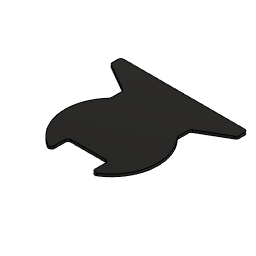
キッカー基板 (Autodesk Fusion 360 design; units mm, degrees)
Autodesk Fusion 360 part; units mm, degrees
note: some values were not read from the file. Set by a fixed rule: which sketch regions a step uses.
(part 1 of 4)
sketch "スケッチ1" plane through (0, 0, 0) normal (0, 0, 1) x (1, 0, 0)
  circle A0 centre (0, 0) radius 104
  line L0 (0, 0) -> (90.0666, 52)
  line L1 (0, 0) -> (104, 0) construction
  dimension "d1" = 208
  dimension "d2" = 30
  constraint coincident A0.centre L0.start
  constraint horizontal L1
  constraint coincident A0 L0.end
  measures "d1" diameter of A0
  measures "d2" angle of L0 L1
extrude "押し出し1" add sketch "スケッチ1" along normal blind 1.5 makes body 1
sketch "スケッチ2" plane through (0, 0, 1.5) normal (0, 0, 1) x (-1, 0, 0)
sketch "スケッチ3" plane through (0, 0, 3) normal (0, 0, 1) x (1, 0, 0)
  circle A0 centre (-65.4951, 21.3591) radius 1.5
  line L0 (-68.4502, 26.2407) -> (-71.2002, 21.4776)
  line L1 (-71.2002, 21.4776) -> (-64.272, 17.4776)
  line L2 (-64.272, 17.4776) -> (-61.522, 22.2407)
  line L3 (-61.522, 22.2407) -> (-68.4502, 26.2407)
sketch "スケッチ4" plane through (0, 0, 3) normal (0, 0, 1) x (1, 0, 0)
  circle A0 centre (65.4951, 21.3591) radius 1.5
  line L0 (71.2002, 21.4776) -> (68.4502, 26.2407)
  line L1 (68.4502, 26.2407) -> (61.522, 22.2407)
  line L2 (61.522, 22.2407) -> (64.272, 17.4776)
  line L3 (64.272, 17.4776) -> (71.2002, 21.4776)
sketch "スケッチ5" plane through (0, 0, 3) normal (0, 0, 1) x (1, 0, 0)
  circle A0 centre (-37.5827, -57.7353) radius 1.5
  line L0 (-43.0628, -59.3263) -> (-39.1737, -63.2153)
  line L1 (-39.1737, -63.2153) -> (-33.5169, -57.5585)
  line L2 (-33.5169, -57.5585) -> (-37.4059, -53.6694)
  line L3 (-37.4059, -53.6694) -> (-43.0628, -59.3263)
sketch "スケッチ6" plane through (0, 0, 3) normal (0, 0, 1) x (1, 0, 0)
  circle A0 centre (51.2451, 46.0409) radius 1.5
  line L0 (56.9502, 46.1593) -> (54.2002, 50.9224)
  line L1 (54.2002, 50.9224) -> (47.272, 46.9224)
  line L2 (47.272, 46.9224) -> (50.022, 42.1593)
  line L3 (50.022, 42.1593) -> (56.9502, 46.1593)
sketch "スケッチ7" plane through (0, 0, 3) normal (0, 0, 1) x (1, 0, 0)
  circle A0 centre (-51.2451, 46.0409) radius 1.5
  line L0 (-54.2002, 50.9224) -> (-56.9502, 46.1593)
  line L1 (-56.9502, 46.1593) -> (-50.022, 42.1593)
  line L2 (-50.022, 42.1593) -> (-47.272, 46.9224)
  line L3 (-47.272, 46.9224) -> (-54.2002, 50.9224)
sketch "スケッチ8" plane through (0, 0, 3) normal (0, 0, 1) x (1, 0, 0)
  circle A0 centre (-57.7353, -37.5827) radius 1.5
  line L0 (-63.2153, -39.1737) -> (-59.3263, -43.0628)
  line L1 (-59.3263, -43.0628) -> (-53.6694, -37.4059)
  line L2 (-53.6694, -37.4059) -> (-57.5585, -33.5169)
  line L3 (-57.5585, -33.5169) -> (-63.2153, -39.1737)
sketch "スケッチ9" plane through (0, 0, 3) normal (0, 0, 1) x (1, 0, 0)
  circle A0 centre (37.5827, -57.7353) radius 1.5
  line L0 (39.1737, -63.2153) -> (43.0628, -59.3263)
  line L1 (43.0628, -59.3263) -> (37.4059, -53.6694)
  line L2 (37.4059, -53.6694) -> (33.5169, -57.5585)
  line L3 (33.5169, -57.5585) -> (39.1737, -63.2153)
sketch "スケッチ10" plane through (0, 0, 3) normal (0, 0, 1) x (1, 0, 0)
  circle A0 centre (57.7353, -37.5827) radius 1.5
  line L0 (59.3263, -43.0628) -> (63.2153, -39.1737)
  line L1 (63.2153, -39.1737) -> (57.5585, -33.5169)
  line L2 (57.5585, -33.5169) -> (53.6694, -37.4059)
  line L3 (53.6694, -37.4059) -> (59.3263, -43.0628)
extrude "押し出し2" cut sketch "スケッチ7" against normal blind 10 contours A0 bodies 1
extrude "押し出し3" cut sketch "スケッチ6" against normal blind 4 contours A0 bodies 1
extrude "押し出し4" cut sketch "スケッチ3" against normal blind 6 contours A0 bodies 1
extrude "押し出し5" cut sketch "スケッチ8" against normal blind 13 contours A0 bodies 1
extrude "押し出し6" cut sketch "スケッチ5" against normal blind 16 contours A0 bodies 1
extrude "押し出し7" cut sketch "スケッチ9" against normal blind 5 contours A0 bodies 1
extrude "押し出し8" cut sketch "スケッチ10" against normal blind 12 contours A0 bodies 1
extrude "押し出し9" cut sketch "スケッチ4" against normal blind 13 contours A0 bodies 1
sketch "スケッチ11" plane through (0, 0, 0) normal (0, 0, -1) x (1, 0, 0)
  circle A0 centre (65.4951, -21.3591) radius 1.5
  circle A1 centre (57.7353, 37.5827) radius 1.5
  circle A2 centre (37.5827, 57.7353) radius 1.5
  circle A3 centre (-37.5827, 57.7353) radius 1.5
  circle A4 centre (-57.7353, 37.5827) radius 1.5
  circle A5 centre (-65.4951, -21.3591) radius 1.5
  circle A6 centre (51.2451, -46.0409) radius 1.5
  circle A7 centre (-51.2451, -46.0409) radius 1.5
  circle A8 centre (0, 0) radius 104
  line L0 (51.2451, -46.0409) -> (65.4951, -21.3591)
  line L1 (-65.4951, -21.3591) -> (-51.2451, -46.0409)
  line L2 (37.5827, 57.7353) -> (57.7353, 37.5827)
  line L3 (-57.7353, 37.5827) -> (-37.5827, 57.7353)
  line L4 (58.3701, -33.7) -> (69.6284, -40.2)
  line L5 (-58.3701, -33.7) -> (-69.6284, -40.2)
  line L6 (47.659, 47.659) -> (56.8514, 56.8514)
  line L7 (-47.659, 47.659) -> (-56.8514, 56.8514)
  line L8 (-56.8514, 56.8514) -> (-35.6382, 78.0646)
  line L9 (-56.8514, 56.8514) -> (-78.0646, 35.6382)
  line L10 (-78.0646, 35.6382) -> (-91.6263, 49.1999)
  line L11 (-35.6382, 78.0646) -> (-49.1999, 91.6263)
  line L12 (56.8514, 56.8514) -> (35.6382, 78.0646)
  line L13 (56.8514, 56.8514) -> (78.0646, 35.6382)
  line L14 (78.0646, 35.6382) -> (91.6263, 49.1999)
  line L15 (35.6382, 78.0646) -> (49.1999, 91.6263)
  line L16 (69.6284, -40.2) -> (84.6284, -14.2192)
  line L17 (84.6284, -14.2192) -> (101.238, -23.8088)
  line L18 (69.6284, -40.2) -> (54.6284, -66.1808)
  line L19 (54.6284, -66.1808) -> (71.238, -75.7703)
  line L20 (-69.6284, -40.2) -> (-54.6284, -66.1808)
  line L21 (-69.6284, -40.2) -> (-84.6284, -14.2192)
  line L22 (-84.6284, -14.2192) -> (-101.238, -23.8088)
  line L23 (-54.6284, -66.1808) -> (-71.238, -75.7703)
  dimension "d26" = 13
  dimension "d27" = 13
  dimension "d28" = 13
  dimension "d29" = 13
  dimension "d30" = 30
  dimension "d31" = 30
  dimension "d32" = 30
  dimension "d33" = 30
  dimension "d34" = 30
  dimension "d35" = 30
  dimension "d36" = 30
  dimension "d37" = 30
  constraint coincident A6.centre L0.start
  constraint coincident A0.centre L0.end
  constraint coincident A5.centre L1.start
  constraint coincident A7.centre L1.end
  constraint coincident A2.centre L2.start
  constraint coincident A1.centre L2.end
  constraint coincident A4.centre L3.start
  constraint coincident A3.centre L3.end
  constraint midpoint L0 L4.start
  constraint perpendicular L0 L4
  constraint midpoint L1 L5.start
  constraint perpendicular L1 L5
  constraint midpoint L2 L6.start
  constraint perpendicular L2 L6
  constraint midpoint L3 L7.start
  constraint perpendicular L3 L7
  constraint perpendicular L7 L8
  constraint perpendicular L7 L9
  constraint coincident A8 L10.end
  constraint perpendicular L9 L10
  constraint coincident A8 L11.end
  constraint perpendicular L8 L11
  constraint perpendicular L6 L12
  constraint perpendicular L6 L13
  constraint coincident A8 L14.end
  constraint perpendicular L13 L14
  constraint coincident A8 L15.end
  constraint perpendicular L12 L15
  constraint perpendicular L4 L16
  constraint coincident A8 L17.end
  constraint perpendicular L16 L17
  constraint perpendicular L4 L18
  constraint coincident A8 L19.end
  constraint perpendicular L18 L19
  constraint perpendicular L5 L20
  constraint perpendicular L5 L21
  constraint coincident A8 L22.end
  constraint perpendicular L21 L22
  constraint coincident A8 L23.end
  constraint perpendicular L20 L23
  measures "d26" distance of L4.start L4.end
  measures "d27" distance of L5.start L5.end
  measures "d28" distance of L6.start L6.end
  measures "d29" distance of L7.start L7.end
  measures "d30" distance of L7.end L8.end
  measures "d31" distance of L7.end L9.end
  measures "d32" distance of L6.end L12.end
  measures "d33" distance of L6.end L13.end
  measures "d34" distance of L4.end L16.end
  measures "d35" distance of L4.end L18.end
  measures "d36" distance of L5.end L20.end
  measures "d37" distance of L5.end L21.end
extrude "押し出し10" cut sketch "スケッチ11" against normal blind 40 contours A8 L12 L13 L14 L15 | A8 L16 L17 L18 L19 | A8 L8 L9 L10 L11 | A8 L20 L21 L22 L23 bodies 1
move_body "移動1" bodies 1 to x (-1, 0, 0) y (0, 1, 0) z (0, 0, -1) at (0, 0, 3)
sketch "スケッチ12" plane through (0, 0, 3) normal (0, 0, 1) x (-1, 0, 0)
  line L0 (35.6382, 78.0646) -> (49.1999, 91.6263)
  arc A0 (49.1999, 91.6263) -> (-49.1999, 91.6263) centre (0, 0) ccw
  line L1 (-49.1999, 91.6263) -> (-35.6382, 78.0646)
  line L2 (-35.6382, 78.0646) -> (-78.0646, 35.6382)
  line L3 (-78.0646, 35.6382) -> (-91.6263, 49.1999)
  arc A1 (-91.6263, 49.1999) -> (-101.238, -23.8088) centre (0, 0) ccw
  line L4 (-101.238, -23.8088) -> (-84.6284, -14.2192)
  line L5 (-84.6284, -14.2192) -> (-54.6284, -66.1808)
  line L6 (-54.6284, -66.1808) -> (-71.238, -75.7703)
  arc A2 (-71.238, -75.7703) -> (71.238, -75.7703) centre (0, 0) ccw
  line L7 (71.238, -75.7703) -> (54.6284, -66.1808)
  line L8 (54.6284, -66.1808) -> (84.6284, -14.2192)
  line L9 (84.6284, -14.2192) -> (101.238, -23.8088)
  arc A3 (101.238, -23.8088) -> (91.6263, 49.1999) centre (0, 0) ccw
  line L10 (91.6263, 49.1999) -> (78.0646, 35.6382)
  line L11 (78.0646, 35.6382) -> (35.6382, 78.0646)
  circle A4 centre (65.4951, -21.3591) radius 1.5
  circle A5 centre (57.7353, 37.5827) radius 1.5
  circle A6 centre (37.5827, 57.7353) radius 1.5
  circle A7 centre (-37.5827, 57.7353) radius 1.5
  circle A8 centre (-57.7353, 37.5827) radius 1.5
  circle A9 centre (-65.4951, -21.3591) radius 1.5
  circle A10 centre (51.2451, -46.0409) radius 1.5
  circle A11 centre (-51.2451, -46.0409) radius 1.5
  line L12 (0, -104) -> (0, -64)
  line L13 (0, -64) -> (-40, -64)
  line L14 (-40, -64) -> (-40, -96)
  line L15 (0, -64) -> (40, -64)
  line L16 (40, -64) -> (40, -96)
  dimension "d40" = 40
  constraint midpoint A2 L12.start
  constraint vertical L12
  constraint perpendicular L12 L13
  constraint coincident A2 L14.end
  constraint perpendicular L13 L14
  constraint perpendicular L14 L15
  constraint coincident A2 L16.end
  constraint perpendicular L15 L16
  measures "d40" distance of L12.start L12.end
extrude "押し出し11" cut sketch "スケッチ12" against normal blind 35 contours A2 L12 L15 L16 | A2 L12 L13 L14 bodies 1
sketch "スケッチ13" plane through (0, 0, 3) normal (0, 0, 1) x (-1, 0, 0)
  line L0 (40, -64) -> (40, -96)
  arc A0 (40, -96) -> (71.238, -75.7703) centre (0, 0) ccw
  line L1 (71.238, -75.7703) -> (54.6284, -66.1808)
  line L2 (54.6284, -66.1808) -> (84.6284, -14.2192)
  line L3 (84.6284, -14.2192) -> (101.238, -23.8088)
  arc A1 (101.238, -23.8088) -> (91.6263, 49.1999) centre (0, 0) ccw
  line L4 (91.6263, 49.1999) -> (78.0646, 35.6382)
  line L5 (78.0646, 35.6382) -> (35.6382, 78.0646)
  line L6 (35.6382, 78.0646) -> (49.1999, 91.6263)
  arc A2 (49.1999, 91.6263) -> (-49.1999, 91.6263) centre (0, 0) ccw
  line L7 (-49.1999, 91.6263) -> (-35.6382, 78.0646)
  line L8 (-35.6382, 78.0646) -> (-78.0646, 35.6382)
  line L9 (-78.0646, 35.6382) -> (-91.6263, 49.1999)
  arc A3 (-91.6263, 49.1999) -> (-101.238, -23.8088) centre (0, 0) ccw
  line L10 (-101.238, -23.8088) -> (-84.6284, -14.2192)
  line L11 (-84.6284, -14.2192) -> (-54.6284, -66.1808)
  line L12 (-54.6284, -66.1808) -> (-71.238, -75.7703)
  arc A4 (-71.238, -75.7703) -> (-40, -96) centre (0, 0) ccw
  line L13 (-40, -96) -> (-40, -64)
  line L14 (-40, -64) -> (40, -64)
  circle A5 centre (65.4951, -21.3591) radius 1.5
  circle A6 centre (57.7353, 37.5827) radius 1.5
  circle A7 centre (37.5827, 57.7353) radius 1.5
  circle A8 centre (-37.5827, 57.7353) radius 1.5
  circle A9 centre (-57.7353, 37.5827) radius 1.5
  circle A10 centre (-65.4951, -21.3591) radius 1.5
  circle A11 centre (51.2451, -46.0409) radius 1.5
  circle A12 centre (-51.2451, -46.0409) radius 1.5
  line L15 (-40, -64) -> (-40, -84)
  line L16 (-40, -84) -> (-61.3188, -84)
  line L17 (40, -84.2208) -> (61.0153, -84.2208)
  dimension "d43" = 20
  constraint coincident L13.end L14.start
  constraint perpendicular L14 L15
  constraint coincident A4 L16.end
  constraint perpendicular L13 L16
  constraint coincident L0 L17.start
  constraint coincident A0 L17.end
  constraint perpendicular L0 L17
  measures "d43" distance of L13.end L15.end
extrude "押し出し12" cut sketch "スケッチ13" against normal blind 18 contours L0 A0 L17 | A4 L13 L16 bodies 1
sketch "スケッチ14" plane through (0, 0, 3) normal (0, 0, 1) x (-1, 0, 0)
  line L0 (40, -84.2208) -> (61.0153, -84.2208)
  arc A0 (61.0153, -84.2208) -> (71.238, -75.7703) centre (0, 0) ccw
  line L1 (71.238, -75.7703) -> (54.6284, -66.1808)
  line L2 (54.6284, -66.1808) -> (84.6284, -14.2192)
  line L3 (84.6284, -14.2192) -> (101.238, -23.8088)
  arc A1 (101.238, -23.8088) -> (91.6263, 49.1999) centre (0, 0) ccw
  line L4 (91.6263, 49.1999) -> (78.0646, 35.6382)
  line L5 (78.0646, 35.6382) -> (35.6382, 78.0646)
  line L6 (35.6382, 78.0646) -> (49.1999, 91.6263)
  arc A2 (49.1999, 91.6263) -> (-49.1999, 91.6263) centre (0, 0) ccw
  line L7 (-49.1999, 91.6263) -> (-35.6382, 78.0646)
  line L8 (-35.6382, 78.0646) -> (-78.0646, 35.6382)
  line L9 (-78.0646, 35.6382) -> (-91.6263, 49.1999)
  arc A3 (-91.6263, 49.1999) -> (-101.238, -23.8088) centre (0, 0) ccw
  line L10 (-101.238, -23.8088) -> (-84.6284, -14.2192)
  line L11 (-84.6284, -14.2192) -> (-54.6284, -66.1808)
  line L12 (-54.6284, -66.1808) -> (-71.238, -75.7703)
  arc A4 (-71.238, -75.7703) -> (-61.3188, -84) centre (0, 0) ccw
  line L13 (-61.3188, -84) -> (-40, -84)
  line L14 (-40, -84) -> (-40, -64)
  line L15 (-40, -64) -> (40, -64)
  line L16 (40, -64) -> (40, -84.2208)
  circle A5 centre (65.4951, -21.3591) radius 1.5
  circle A6 centre (57.7353, 37.5827) radius 1.5
  circle A7 centre (37.5827, 57.7353) radius 1.5
  circle A8 centre (-37.5827, 57.7353) radius 1.5
  circle A9 centre (-57.7353, 37.5827) radius 1.5
  circle A10 centre (-65.4951, -21.3591) radius 1.5
  circle A11 centre (51.2451, -46.0409) radius 1.5
  circle A12 centre (-51.2451, -46.0409) radius 1.5
  circle A13 centre (0, 0) radius 50
  constraint coincident A0.centre A1.centre
extrude "押し出し13" cut sketch "スケッチ14" against normal blind 30 contours A13 bodies 1
sketch "スケッチ15" plane through (0, 0, 3) normal (0, 0, 1) x (-1, 0, 0)
  circle A0 centre (0, 0) radius 50
  line L0 (40, -84.2208) -> (61.0153, -84.2208)
  arc A1 (61.0153, -84.2208) -> (71.238, -75.7703) centre (0, 0) ccw
  line L1 (71.238, -75.7703) -> (54.6284, -66.1808)
  line L2 (54.6284, -66.1808) -> (84.6284, -14.2192)
  line L3 (84.6284, -14.2192) -> (101.238, -23.8088)
  arc A2 (101.238, -23.8088) -> (91.6263, 49.1999) centre (0, 0) ccw
  line L4 (91.6263, 49.1999) -> (78.0646, 35.6382)
  line L5 (78.0646, 35.6382) -> (35.6382, 78.0646)
  line L6 (35.6382, 78.0646) -> (49.1999, 91.6263)
  arc A3 (49.1999, 91.6263) -> (-49.1999, 91.6263) centre (0, 0) ccw
  line L7 (-49.1999, 91.6263) -> (-35.6382, 78.0646)
  line L8 (-35.6382, 78.0646) -> (-78.0646, 35.6382)
  line L9 (-78.0646, 35.6382) -> (-91.6263, 49.1999)
  arc A4 (-91.6263, 49.1999) -> (-101.238, -23.8088) centre (0, 0) ccw
  line L10 (-101.238, -23.8088) -> (-84.6284, -14.2192)
  line L11 (-84.6284, -14.2192) -> (-54.6284, -66.1808)
  line L12 (-54.6284, -66.1808) -> (-71.238, -75.7703)
  arc A5 (-71.238, -75.7703) -> (-61.3188, -84) centre (0, 0) ccw
  line L13 (-61.3188, -84) -> (-40, -84)
  line L14 (-40, -84) -> (-40, -64)
  line L15 (-40, -64) -> (40, -64)
  line L16 (40, -64) -> (40, -84.2208)
  circle A6 centre (65.4951, -21.3591) radius 1.5
  circle A7 centre (57.7353, 37.5827) radius 1.5
  circle A8 centre (37.5827, 57.7353) radius 1.5
  circle A9 centre (-37.5827, 57.7353) radius 1.5
  circle A10 centre (-57.7353, 37.5827) radius 1.5
  circle A11 centre (-65.4951, -21.3591) radius 1.5
  circle A12 centre (51.2451, -46.0409) radius 1.5
  circle A13 centre (-51.2451, -46.0409) radius 1.5
  circle A14 centre (0, 0) radius 42
  dimension "d48" = 84
  constraint coincident A0.centre A1.centre
  measures "d48" diameter of A14
extrude "押し出し14" add sketch "スケッチ15" against normal blind 1.5 separate body contours A14 makes body 2
sketch "スケッチ16" plane through (0, 0, 3) normal (0, 0, 1) x (-1, 0, 0)
  circle A0 centre (0, 0) radius 42
  circle A1 centre (0, 0) radius 37
  dimension "d51" = 74
  constraint concentric A0 A1
  measures "d51" diameter of A1
extrude "押し出し15" cut sketch "スケッチ16" against normal blind 25 contours A1 bodies 2
sketch "スケッチ17" plane through (0, 0, 3) normal (0, 0, 1) x (-1, 0, 0)
  circle A0 centre (0, 0) radius 50
  line L0 (40, -84.2208) -> (61.0153, -84.2208)
  arc A1 (61.0153, -84.2208) -> (71.238, -75.7703) centre (0, 0) ccw
  line L1 (71.238, -75.7703) -> (54.6284, -66.1808)
  line L2 (54.6284, -66.1808) -> (84.6284, -14.2192)
  line L3 (84.6284, -14.2192) -> (101.238, -23.8088)
  arc A2 (101.238, -23.8088) -> (91.6263, 49.1999) centre (0, 0) ccw
  line L4 (91.6263, 49.1999) -> (78.0646, 35.6382)
  line L5 (78.0646, 35.6382) -> (35.6382, 78.0646)
  line L6 (35.6382, 78.0646) -> (49.1999, 91.6263)
  arc A3 (49.1999, 91.6263) -> (-49.1999, 91.6263) centre (0, 0) ccw
  line L7 (-49.1999, 91.6263) -> (-35.6382, 78.0646)
  line L8 (-35.6382, 78.0646) -> (-78.0646, 35.6382)
  line L9 (-78.0646, 35.6382) -> (-91.6263, 49.1999)
  arc A4 (-91.6263, 49.1999) -> (-101.238, -23.8088) centre (0, 0) ccw
  line L10 (-101.238, -23.8088) -> (-84.6284, -14.2192)
  line L11 (-84.6284, -14.2192) -> (-54.6284, -66.1808)
  line L12 (-54.6284, -66.1808) -> (-71.238, -75.7703)
  arc A5 (-71.238, -75.7703) -> (-61.3188, -84) centre (0, 0) ccw
  line L13 (-61.3188, -84) -> (-40, -84)
  line L14 (-40, -84) -> (-40, -64)
  line L15 (-40, -64) -> (40, -64)
  line L16 (40, -64) -> (40, -84.2208)
  circle A6 centre (65.4951, -21.3591) radius 1.5
  circle A7 centre (57.7353, 37.5827) radius 1.5
  circle A8 centre (37.5827, 57.7353) radius 1.5
  circle A9 centre (-37.5827, 57.7353) radius 1.5
  circle A10 centre (-57.7353, 37.5827) radius 1.5
  circle A11 centre (-65.4951, -21.3591) radius 1.5
  circle A12 centre (51.2451, -46.0409) radius 1.5
  circle A13 centre (-51.2451, -46.0409) radius 1.5
  line L17 (0, -64) -> (0, -58)
  line L18 (0, -58) -> (-40, -58)
  line L19 (-40, -58) -> (-40, -50)
  line L20 (-40, -50) -> (0, -50)
  line L21 (0, -58) -> (40, -58)
  line L22 (40, -58) -> (40, -50)
  line L23 (40, -50) -> (0, -50)
  line L24 (-4, -50.1) -> (-4, -50)
  constraint midpoint L15 L17.start
  constraint perpendicular L15 L17
  constraint perpendicular L17 L18
  constraint perpendicular L18 L19
  constraint coincident A0 L20.end
  constraint tangent A0 L20
  constraint perpendicular L17 L21
  constraint perpendicular L21 L22
  constraint tangent A0 L23
  constraint coincident L20 L24.end
  constraint perpendicular L20 L24
extrude "押し出し16" cut sketch "スケッチ17" against normal blind 13 contours L18 L19 L20 L21 L22 L23 bodies 1
sketch "スケッチ18" plane through (0, 0, 3) normal (0, 0, 1) x (-1, 0, 0)
  circle A0 centre (-51.2451, -46.0409) radius 1.5
  circle A1 centre (51.2451, -46.0409) radius 1.5
  circle A2 centre (-65.4951, -21.3591) radius 1.5
  circle A3 centre (-57.7353, 37.5827) radius 1.5
  circle A4 centre (-37.5827, 57.7353) radius 1.5
  circle A5 centre (37.5827, 57.7353) radius 1.5
  circle A6 centre (57.7353, 37.5827) radius 1.5
  circle A7 centre (65.4951, -21.3591) radius 1.5
  line L0 (40, -84.2208) -> (61.0153, -84.2208)
  arc A8 (61.0153, -84.2208) -> (71.238, -75.7703) centre (0, 0) ccw
  line L1 (71.238, -75.7703) -> (54.6284, -66.1808)
  line L2 (54.6284, -66.1808) -> (84.6284, -14.2192)
  line L3 (84.6284, -14.2192) -> (101.238, -23.8088)
  arc A9 (101.238, -23.8088) -> (91.6263, 49.1999) centre (0, 0) ccw
  line L4 (91.6263, 49.1999) -> (78.0646, 35.6382)
  line L5 (78.0646, 35.6382) -> (35.6382, 78.0646)
  line L6 (35.6382, 78.0646) -> (49.1999, 91.6263)
  arc A10 (49.1999, 91.6263) -> (-49.1999, 91.6263) centre (0, 0) ccw
  line L7 (-49.1999, 91.6263) -> (-35.6382, 78.0646)
  line L8 (-35.6382, 78.0646) -> (-78.0646, 35.6382)
  line L9 (-78.0646, 35.6382) -> (-91.6263, 49.1999)
  arc A11 (-91.6263, 49.1999) -> (-101.238, -23.8088) centre (0, 0) ccw
  line L10 (-101.238, -23.8088) -> (-84.6284, -14.2192)
  line L11 (-84.6284, -14.2192) -> (-54.6284, -66.1808)
  line L12 (-54.6284, -66.1808) -> (-71.238, -75.7703)
  arc A12 (-71.238, -75.7703) -> (-61.3188, -84) centre (0, 0) ccw
  line L13 (-61.3188, -84) -> (-40, -84)
  line L14 (-40, -84) -> (-40, -64)
  line L15 (-40, -64) -> (40, -64)
  line L16 (40, -64) -> (40, -84.2208)
  circle A13 centre (0, 0) radius 50
  line L17 (0, -50) -> (40, -50)
  line L18 (40, -50) -> (40, -58)
  line L19 (40, -58) -> (-40, -58)
  line L20 (-40, -58) -> (-40, -50)
  line L21 (-40, -50) -> (0, -50)
  circle A14 centre (0, 0) radius 45
  circle A15 centre (0, 0) radius 371.5
  dimension "d56" = 743
  constraint coincident A8.centre A9.centre
  constraint concentric A8 A15
  measures "d56" diameter of A15
extrude "押し出し17" add sketch "スケッチ18" against normal blind 1.5 contours A13 bodies 1
sketch "スケッチ19" plane through (0, 0, 3) normal (0, 0, 1) x (-1, 0, 0)
  circle A0 centre (0, 0) radius 45
  circle A1 centre (-51.2451, -46.0409) radius 1.5
  circle A2 centre (51.2451, -46.0409) radius 1.5
  circle A3 centre (-65.4951, -21.3591) radius 1.5
  circle A4 centre (-57.7353, 37.5827) radius 1.5
  circle A5 centre (-37.5827, 57.7353) radius 1.5
  circle A6 centre (37.5827, 57.7353) radius 1.5
  circle A7 centre (57.7353, 37.5827) radius 1.5
  circle A8 centre (65.4951, -21.3591) radius 1.5
  line L0 (40, -84.2208) -> (61.0153, -84.2208)
  arc A9 (61.0153, -84.2208) -> (71.238, -75.7703) centre (0, 0) ccw
  line L1 (71.238, -75.7703) -> (54.6284, -66.1808)
  line L2 (54.6284, -66.1808) -> (84.6284, -14.2192)
  line L3 (84.6284, -14.2192) -> (101.238, -23.8088)
  arc A10 (101.238, -23.8088) -> (91.6263, 49.1999) centre (0, 0) ccw
  line L4 (91.6263, 49.1999) -> (78.0646, 35.6382)
  line L5 (78.0646, 35.6382) -> (35.6382, 78.0646)
  line L6 (35.6382, 78.0646) -> (49.1999, 91.6263)
  arc A11 (49.1999, 91.6263) -> (-49.1999, 91.6263) centre (0, 0) ccw
  line L7 (-49.1999, 91.6263) -> (-35.6382, 78.0646)
  line L8 (-35.6382, 78.0646) -> (-78.0646, 35.6382)
  line L9 (-78.0646, 35.6382) -> (-91.6263, 49.1999)
  arc A12 (-91.6263, 49.1999) -> (-101.238, -23.8088) centre (0, 0) ccw
  line L10 (-101.238, -23.8088) -> (-84.6284, -14.2192)
  line L11 (-84.6284, -14.2192) -> (-54.6284, -66.1808)
  line L12 (-54.6284, -66.1808) -> (-71.238, -75.7703)
  arc A13 (-71.238, -75.7703) -> (-61.3188, -84) centre (0, 0) ccw
  line L13 (-61.3188, -84) -> (-40, -84)
  line L14 (-40, -84) -> (-40, -64)
  line L15 (-40, -64) -> (40, -64)
  line L16 (40, -64) -> (40, -84.2208)
  line L17 (0, -50) -> (40, -50)
  line L18 (40, -50) -> (40, -58)
  line L19 (40, -58) -> (-40, -58)
  line L20 (-40, -58) -> (-40, -50)
  line L21 (-40, -50) -> (0, -50)
  circle A14 centre (0, 0) radius 37
  circle A15 centre (0, 0) radius 32
  constraint coincident A0.centre A9.centre
  constraint concentric A0 A15
extrude "押し出し18" cut sketch "スケッチ19" against normal blind 14 contours A0 bodies 2
sketch "スケッチ20" plane through (0, 0, 3) normal (0, 0, 1) x (-1, 0, 0)
  circle A0 centre (0, 0) radius 45
  circle A1 centre (-51.2451, -46.0409) radius 1.5
  circle A2 centre (51.2451, -46.0409) radius 1.5
  circle A3 centre (-65.4951, -21.3591) radius 1.5
  circle A4 centre (-57.7353, 37.5827) radius 1.5
  circle A5 centre (-37.5827, 57.7353) radius 1.5
  circle A6 centre (37.5827, 57.7353) radius 1.5
  circle A7 centre (57.7353, 37.5827) radius 1.5
  circle A8 centre (65.4951, -21.3591) radius 1.5
  line L0 (40, -84.2208) -> (61.0153, -84.2208)
  arc A9 (61.0153, -84.2208) -> (71.238, -75.7703) centre (0, 0) ccw
  line L1 (71.238, -75.7703) -> (54.6284, -66.1808)
  line L2 (54.6284, -66.1808) -> (84.6284, -14.2192)
  line L3 (84.6284, -14.2192) -> (101.238, -23.8088)
  arc A10 (101.238, -23.8088) -> (91.6263, 49.1999) centre (0, 0) ccw
  line L4 (91.6263, 49.1999) -> (78.0646, 35.6382)
  line L5 (78.0646, 35.6382) -> (35.6382, 78.0646)
  line L6 (35.6382, 78.0646) -> (49.1999, 91.6263)
  arc A11 (49.1999, 91.6263) -> (-49.1999, 91.6263) centre (0, 0) ccw
  line L7 (-49.1999, 91.6263) -> (-35.6382, 78.0646)
  line L8 (-35.6382, 78.0646) -> (-78.0646, 35.6382)
  line L9 (-78.0646, 35.6382) -> (-91.6263, 49.1999)
  arc A12 (-91.6263, 49.1999) -> (-101.238, -23.8088) centre (0, 0) ccw
  line L10 (-101.238, -23.8088) -> (-84.6284, -14.2192)
  line L11 (-84.6284, -14.2192) -> (-54.6284, -66.1808)
  line L12 (-54.6284, -66.1808) -> (-71.238, -75.7703)
  arc A13 (-71.238, -75.7703) -> (-61.3188, -84) centre (0, 0) ccw
  line L13 (-61.3188, -84) -> (-40, -84)
  line L14 (-40, -84) -> (-40, -64)
  line L15 (-40, -64) -> (40, -64)
  line L16 (40, -64) -> (40, -84.2208)
  line L17 (0, -50) -> (40, -50)
  line L18 (40, -50) -> (40, -58)
  line L19 (40, -58) -> (-40, -58)
  line L20 (-40, -58) -> (-40, -50)
  line L21 (-40, -50) -> (0, -50)
  circle A14 centre (0, 0) radius 32
  circle A15 centre (0, 0) radius 37
  dimension "d61" = 64
  dimension "d62" = 74
  constraint coincident A0.centre A9.centre
  constraint concentric A0 A15
  measures "d61" diameter of A14
  measures "d62" diameter of A15
extrude "押し出し19" add sketch "スケッチ20" against normal blind 1.5 contours A15 bodies 2
sketch "スケッチ21" plane through (0, 0, 3) normal (0, 0, 1) x (-1, 0, 0)
  circle A0 centre (0, 0) radius 45
  circle A1 centre (-51.2451, -46.0409) radius 1.5
  circle A2 centre (51.2451, -46.0409) radius 1.5
  circle A3 centre (-65.4951, -21.3591) radius 1.5
  circle A4 centre (-57.7353, 37.5827) radius 1.5
  circle A5 centre (-37.5827, 57.7353) radius 1.5
  circle A6 centre (37.5827, 57.7353) radius 1.5
  circle A7 centre (57.7353, 37.5827) radius 1.5
  circle A8 centre (65.4951, -21.3591) radius 1.5
  line L0 (40, -84.2208) -> (61.0153, -84.2208)
  arc A9 (61.0153, -84.2208) -> (71.238, -75.7703) centre (0, 0) ccw
  line L1 (71.238, -75.7703) -> (54.6284, -66.1808)
  line L2 (54.6284, -66.1808) -> (84.6284, -14.2192)
  line L3 (84.6284, -14.2192) -> (101.238, -23.8088)
  arc A10 (101.238, -23.8088) -> (91.6263, 49.1999) centre (0, 0) ccw
  line L4 (91.6263, 49.1999) -> (78.0646, 35.6382)
  line L5 (78.0646, 35.6382) -> (35.6382, 78.0646)
  line L6 (35.6382, 78.0646) -> (49.1999, 91.6263)
  arc A11 (49.1999, 91.6263) -> (-49.1999, 91.6263) centre (0, 0) ccw
  line L7 (-49.1999, 91.6263) -> (-35.6382, 78.0646)
  line L8 (-35.6382, 78.0646) -> (-78.0646, 35.6382)
  line L9 (-78.0646, 35.6382) -> (-91.6263, 49.1999)
  arc A12 (-91.6263, 49.1999) -> (-101.238, -23.8088) centre (0, 0) ccw
  line L10 (-101.238, -23.8088) -> (-84.6284, -14.2192)
  line L11 (-84.6284, -14.2192) -> (-54.6284, -66.1808)
  line L12 (-54.6284, -66.1808) -> (-71.238, -75.7703)
  arc A13 (-71.238, -75.7703) -> (-61.3188, -84) centre (0, 0) ccw
  line L13 (-61.3188, -84) -> (-40, -84)
  line L14 (-40, -84) -> (-40, -64)
  line L15 (-40, -64) -> (40, -64)
  line L16 (40, -64) -> (40, -84.2208)
  line L17 (0, -50) -> (40, -50)
  line L18 (40, -50) -> (40, -58)
  line L19 (40, -58) -> (-40, -58)
  line L20 (-40, -58) -> (-40, -50)
  line L21 (-40, -50) -> (0, -50)
  line L22 (0, -47) -> (-4, -47)
  line L23 (0, -47) -> (4, -47)
  line L24 (4, -47) -> (4, -50)
  line L25 (-4, -47) -> (-4, -50)
  line L26 (-4, -47) -> (-4, -44.8219)
  line L27 (4, -47) -> (4, -44.8219)
  dimension "d65" = 4
  dimension "d66" = 4
  constraint parallel L17 L22
  constraint parallel L22 L23
  constraint coincident L17 L24.end
  constraint perpendicular L17 L24
  constraint coincident L21 L25.end
  constraint perpendicular L21 L25
  constraint coincident A0 L26.end
  constraint perpendicular L22 L26
  constraint coincident A0 L27.end
  constraint perpendicular L23 L27
  measures "d65" distance of L22.start L22.end
  measures "d66" distance of L22.start L23.end
extrude "押し出し20" cut sketch "スケッチ21" against normal blind 7 contours A0 L22 L23 L26 L27 | L17 L21 L22 L23 L24 L25 bodies 1
sketch "スケッチ22" plane through (0, 0, 3) normal (0, 0, 1) x (-1, 0, 0)
  line L0 (40, -84.2208) -> (61.0153, -84.2208)
  arc A0 (61.0153, -84.2208) -> (71.238, -75.7703) centre (0, 0) ccw
  line L1 (71.238, -75.7703) -> (54.6284, -66.1808)
  line L2 (54.6284, -66.1808) -> (84.6284, -14.2192)
  line L3 (84.6284, -14.2192) -> (101.238, -23.8088)
  arc A1 (101.238, -23.8088) -> (91.6263, 49.1999) centre (0, 0) ccw
  line L4 (91.6263, 49.1999) -> (78.0646, 35.6382)
  line L5 (78.0646, 35.6382) -> (35.6382, 78.0646)
  line L6 (35.6382, 78.0646) -> (49.1999, 91.6263)
  arc A2 (49.1999, 91.6263) -> (-49.1999, 91.6263) centre (0, 0) ccw
  line L7 (-49.1999, 91.6263) -> (-35.6382, 78.0646)
  line L8 (-35.6382, 78.0646) -> (-78.0646, 35.6382)
  line L9 (-78.0646, 35.6382) -> (-91.6263, 49.1999)
  arc A3 (-91.6263, 49.1999) -> (-101.238, -23.8088) centre (0, 0) ccw
  line L10 (-101.238, -23.8088) -> (-84.6284, -14.2192)
  line L11 (-84.6284, -14.2192) -> (-54.6284, -66.1808)
  line L12 (-54.6284, -66.1808) -> (-71.238, -75.7703)
  arc A4 (-71.238, -75.7703) -> (-61.3188, -84) centre (0, 0) ccw
  line L13 (-61.3188, -84) -> (-40, -84)
  line L14 (-40, -84) -> (-40, -64)
  line L15 (-40, -64) -> (40, -64)
  line L16 (40, -64) -> (40, -84.2208)
  circle A5 centre (65.4951, -21.3591) radius 1.5
  circle A6 centre (57.7353, 37.5827) radius 1.5
  circle A7 centre (37.5827, 57.7353) radius 1.5
  circle A8 centre (-37.5827, 57.7353) radius 1.5
  circle A9 centre (-57.7353, 37.5827) radius 1.5
  circle A10 centre (-65.4951, -21.3591) radius 1.5
  circle A11 centre (51.2451, -46.0409) radius 1.5
  circle A12 centre (-51.2451, -46.0409) radius 1.5
  line L17 (-4, -50) -> (-4, -47)
  line L18 (-4, -47) -> (-4, -44.8219)
  arc A13 (4, -44.8219) -> (-4, -44.8219) centre (0, 0) ccw
  line L19 (4, -44.8219) -> (4, -50)
  line L20 (4, -50) -> (40, -50)
  line L21 (40, -50) -> (40, -58)
  line L22 (40, -58) -> (-40, -58)
  line L23 (-40, -58) -> (-40, -50)
  line L24 (-40, -50) -> (-4, -50)
  line L25 (-75, 0) -> (-75, -4)
  line L26 (-75, -4) -> (-44.8219, -4)
  line L27 (-75, -4) -> (-101, -4)
  line L28 (-75, 0) -> (-75, 4)
  line L29 (-75, 4) -> (-44.8219, 4)
  line L30 (-75, 4) -> (-102, 4)
  line L31 (52.8219, 0) -> (52.8219, -4)
  line L32 (52.8219, -4) -> (44.8219, -4)
  line L33 (52.8219, -4) -> (101, -4)
  line L34 (52.8219, 0) -> (52.8219, 4)
  line L35 (52.8219, 4) -> (44.8219, 4)
  line L36 (52.8219, 4) -> (102, 4)
  line L37 (0, 65) -> (-4, 65)
  line L38 (-4, 65) -> (-4, 44.8219)
  line L39 (-4, 65) -> (-4, 102)
  line L40 (0, 65) -> (4, 65)
  line L41 (4, 65) -> (4, 44.8219)
  line L42 (4, 65) -> (4, 102)
  circle A14 centre (0, 0) radius 99
  dimension "d69" = 4
  dimension "d70" = 4
  dimension "d71" = 198
  constraint vertical L25
  constraint coincident A13 L26.end
  constraint perpendicular L25 L26
  constraint perpendicular L25 L27
  constraint perpendicular L27 L28
  constraint coincident A13 L29.end
  constraint perpendicular L28 L29
  constraint perpendicular L28 L30
  constraint perpendicular L30 L31
  constraint coincident A13 L32.end
  constraint perpendicular L31 L32
  constraint perpendicular L31 L33
  constraint perpendicular L33 L34
  constraint coincident A13 L35.end
  constraint perpendicular L34 L35
  constraint perpendicular L34 L36
  constraint parallel L36 L37
  constraint coincident A13 L38.end
  constraint perpendicular L36 L38
  constraint perpendicular L37 L39
  constraint perpendicular L39 L40
  constraint coincident A13 L41.end
  constraint perpendicular L40 L41
  constraint perpendicular L40 L42
  constraint coincident A0.centre A1.centre
  measures "d69" distance of L37.start L37.end
  measures "d70" distance of L37.start L40.end
  measures "d71" diameter of A14
extrude "押し出し21" cut sketch "スケッチ22" against normal blind 15 contours L31 L33 L34 L36 A14 | L25 L27 L28 L30 A14 | A13 L31 L32 L34 L35 | A13 L25 L26 L28 L29 | L37 L39 L40 L42 A14 | A13 L37 L38 L40 L41 bodies 1
sketch "スケッチ23" plane through (0, 0, 3) normal (0, 0, 1) x (-1, 0, 0)
  circle A0 centre (0, 0) radius 32
  circle A1 centre (0, 0) radius 37
  line L0 (0, 0) -> (-33, -32)
  line L1 (0, 0) -> (34.6979, 33.6464)
  line L2 (0, 0) -> (32.1657, -33.1709)
  line L3 (0, 0) -> (-35.118, 36.2154)
  line L4 (-29.7936, -28.8908) -> (-31.534, -27.096)
  line L5 (-29.7936, -28.8908) -> (-28.0532, -30.6855)
  line L6 (-28.0532, -30.6855) -> (-31.0569, -33.5982)
  line L7 (-31.534, -27.096) -> (-35.2356, -30.6855)
  line L8 (-31.534, -27.096) -> (-27.7794, -23.4552)
  line L9 (-28.0532, -30.6855) -> (-24.0023, -26.7574)
  line L10 (28.776, -29.6752) -> (26.9812, -31.4156)
  line L11 (28.776, -29.6752) -> (30.5707, -27.9348)
  line L12 (30.5707, -27.9348) -> (33.6846, -31.146)
  line L13 (26.9812, -31.4156) -> (30.5707, -35.1172)
  line L14 (30.5707, -27.9348) -> (26.9812, -24.2332)
  line L15 (26.9812, -31.4156) -> (23.0883, -27.401)
  line L16 (-28.6584, 29.554) -> (-30.4532, 27.8136)
  line L17 (-28.6584, 29.554) -> (-26.8637, 31.2944)
  line L18 (-30.4532, 27.8136) -> (-27.4933, 24.7612)
  line L19 (-30.4532, 27.8136) -> (-33.182, 30.6278)
  line L20 (-26.8637, 31.2944) -> (-23.9038, 28.242)
  line L21 (-26.8637, 31.2944) -> (-30.0313, 34.5609)
  line L22 (29.1245, 28.242) -> (27.3842, 30.0367)
  line L23 (29.1245, 28.242) -> (30.8649, 26.4472)
  line L24 (30.8649, 26.4472) -> (28.242, 23.9038)
  line L25 (27.3842, 30.0367) -> (24.7612, 27.4933)
  line L26 (27.3842, 30.0367) -> (30.7309, 33.282)
  line L27 (30.8649, 26.4472) -> (34.5666, 30.0367)
  circle A2 centre (0, 0) radius 45
  dimension "d74" = 2.5
  dimension "d75" = 2.5
  dimension "d76" = 2.5
  dimension "d77" = 2.5
  dimension "d78" = 2.5
  dimension "d79" = 2.5
  dimension "d80" = 2.5
  dimension "d81" = 2.5
  constraint coincident A0.centre A1.centre
  constraint parallel L0 L1
  constraint perpendicular L0 L2
  constraint perpendicular L1 L3
  constraint coincident L0 L4.start
  constraint perpendicular L0 L4
  constraint perpendicular L0 L5
  constraint perpendicular L5 L6
  constraint perpendicular L4 L7
  constraint perpendicular L4 L8
  constraint perpendicular L5 L9
  constraint coincident L2 L10.start
  constraint perpendicular L2 L10
  constraint perpendicular L2 L11
  constraint perpendicular L11 L12
  constraint perpendicular L10 L13
  constraint perpendicular L11 L14
  constraint perpendicular L10 L15
  constraint coincident L3 L16.start
  constraint perpendicular L3 L16
  constraint perpendicular L3 L17
  constraint coincident A1 L18.end
  constraint perpendicular L16 L18
  constraint perpendicular L16 L19
  constraint coincident A1 L20.end
  constraint perpendicular L17 L20
  constraint perpendicular L17 L21
  constraint coincident L1 L22.start
  constraint perpendicular L1 L22
  constraint perpendicular L1 L23
  constraint coincident A1 L24.end
  constraint perpendicular L23 L24
  constraint coincident A1 L25.end
  constraint perpendicular L22 L25
  constraint perpendicular L22 L26
  constraint perpendicular L23 L27
  measures "d74" distance of L4.start L4.end
  measures "d75" distance of L4.start L5.end
  measures "d76" distance of L10.start L10.end
  measures "d77" distance of L10.start L11.end
  measures "d78" distance of L16.start L16.end
  measures "d79" distance of L16.start L17.end
  measures "d80" distance of L22.start L22.end
  measures "d81" distance of L22.start L23.end
extrude "押し出し22" add sketch "スケッチ23" against normal blind 1.5 contours A1 L1 L23 L24 | A1 L1 L22 L25 | A1 L2 L10 L15 | A1 L2 L11 L14 | A1 L3 L17 L20 | A1 L3 L16 L18 | L1 L22 L26 A2 | L1 L23 L27 A2 | A1 L0 L4 L8 | A1 L0 L5 L9 | L2 L11 L12 A2 | L2 L10 L13 A2 | L3 L16 L19 A2 | L3 L17 L21 A2 | L0 L5 L6 A2 | L0 L4 L7 A2 bodies 1 2
sketch "スケッチ24" plane through (0, 0, 3) normal (0, 0, 1) x (-1, 0, 0)
  arc A0 (44.8219, 4) -> (33.996, 29.4834) centre (0, 0) ccw
  line L0 (44.8219, 4) -> (98.9192, 4)
  arc A1 (98.9192, -4) -> (98.9192, 4) centre (0, 0) ccw
  line L1 (98.9192, -4) -> (44.8219, -4)
  arc A2 (33.0729, -30.5153) -> (44.8219, -4) centre (0, 0) ccw
  line L2 (33.0729, -30.5153) -> (27.4933, -24.7612)
  arc A3 (27.4933, -24.7612) -> (28.242, 23.9038) centre (0, 0) ccw
  line L3 (28.242, 23.9038) -> (33.996, 29.4834)
  arc A4 (4, -44.8219) -> (29.4834, -33.996) centre (0, 0) ccw
  line L4 (4, -44.8219) -> (4, -50)
  line L5 (4, -50) -> (40, -50)
  line L6 (40, -50) -> (40, -58)
  line L7 (40, -58) -> (-40, -58)
  line L8 (-40, -58) -> (-40, -50)
  line L9 (-40, -50) -> (-4, -50)
  line L10 (-4, -50) -> (-4, -47)
  line L11 (-4, -47) -> (-4, -44.8219)
  arc A5 (-30.5153, -33.0729) -> (-4, -44.8219) centre (0, 0) ccw
  line L12 (-30.5153, -33.0729) -> (-24.7612, -27.4933)
  arc A6 (-24.7612, -27.4933) -> (23.9038, -28.242) centre (0, 0) ccw
  line L13 (23.9038, -28.242) -> (29.4834, -33.996)
  line L14 (30.5153, 33.0729) -> (24.7612, 27.4933)
  arc A7 (24.7612, 27.4933) -> (-23.9038, 28.242) centre (0, 0) ccw
  line L15 (-23.9038, 28.242) -> (-29.4834, 33.996)
  arc A8 (-4, 44.8219) -> (-29.4834, 33.996) centre (0, 0) ccw
  line L16 (-4, 44.8219) -> (-4, 98.9192)
  arc A9 (4, 98.9192) -> (-4, 98.9192) centre (0, 0) ccw
  line L17 (4, 98.9192) -> (4, 44.8219)
  arc A10 (30.5153, 33.0729) -> (4, 44.8219) centre (0, 0) ccw
  circle A11 centre (0, 0) radius 32
  line L18 (-33.0729, 30.5153) -> (-27.4933, 24.7612)
  arc A12 (-27.4933, 24.7612) -> (-28.242, -23.9038) centre (0, 0) ccw
  line L19 (-28.242, -23.9038) -> (-33.996, -29.4834)
  arc A13 (-44.8219, -4) -> (-33.996, -29.4834) centre (0, 0) ccw
  line L20 (-44.8219, -4) -> (-98.9192, -4)
  arc A14 (-98.9192, 4) -> (-98.9192, -4) centre (0, 0) ccw
  line L21 (-98.9192, 4) -> (-44.8219, 4)
  arc A15 (-33.0729, 30.5153) -> (-44.8219, 4) centre (0, 0) ccw
  circle A16 centre (-51.2451, -46.0409) radius 1.5
  circle A17 centre (51.2451, -46.0409) radius 1.5
  circle A18 centre (-65.4951, -21.3591) radius 1.5
  circle A19 centre (-57.7353, 37.5827) radius 1.5
  circle A20 centre (-37.5827, 57.7353) radius 1.5
  circle A21 centre (37.5827, 57.7353) radius 1.5
  circle A22 centre (57.7353, 37.5827) radius 1.5
  circle A23 centre (65.4951, -21.3591) radius 1.5
  line L22 (40, -84.2208) -> (61.0153, -84.2208)
  arc A24 (61.0153, -84.2208) -> (71.238, -75.7703) centre (0, 0) ccw
  line L23 (71.238, -75.7703) -> (54.6284, -66.1808)
  line L24 (54.6284, -66.1808) -> (84.6284, -14.2192)
  line L25 (84.6284, -14.2192) -> (101.238, -23.8088)
  arc A25 (101.238, -23.8088) -> (91.6263, 49.1999) centre (0, 0) ccw
  line L26 (91.6263, 49.1999) -> (78.0646, 35.6382)
  line L27 (78.0646, 35.6382) -> (35.6382, 78.0646)
  line L28 (35.6382, 78.0646) -> (49.1999, 91.6263)
  arc A26 (49.1999, 91.6263) -> (-49.1999, 91.6263) centre (0, 0) ccw
  line L29 (-49.1999, 91.6263) -> (-35.6382, 78.0646)
  line L30 (-35.6382, 78.0646) -> (-78.0646, 35.6382)
  line L31 (-78.0646, 35.6382) -> (-91.6263, 49.1999)
  arc A27 (-91.6263, 49.1999) -> (-101.238, -23.8088) centre (0, 0) ccw
  line L32 (-101.238, -23.8088) -> (-84.6284, -14.2192)
  line L33 (-84.6284, -14.2192) -> (-54.6284, -66.1808)
  line L34 (-54.6284, -66.1808) -> (-71.238, -75.7703)
  arc A28 (-71.238, -75.7703) -> (-61.3188, -84) centre (0, 0) ccw
  line L35 (-61.3188, -84) -> (-40, -84)
  line L36 (-40, -84) -> (-40, -64)
  line L37 (-40, -64) -> (40, -64)
  line L38 (40, -64) -> (40, -84.2208)
  line L39 (-69.6284, -40.2) -> (-65.2983, -37.7)
  line L40 (-56.8514, 56.8514) -> (-53.3159, 53.3159)
  line L41 (56.8514, 56.8514) -> (53.3159, 53.3159)
  line L42 (69.6284, -40.2) -> (65.2983, -37.7)
  circle A29 centre (-51.2451, -46.0409) radius 2.5
  circle A30 centre (-65.4951, -21.3591) radius 2.5
  circle A31 centre (-57.7353, 37.5827) radius 2.5
  circle A32 centre (-37.5827, 57.7353) radius 2.5
  circle A33 centre (37.5827, 57.7353) radius 2.5
  circle A34 centre (57.7353, 37.5827) radius 2.5
  circle A35 centre (65.4951, -21.3591) radius 2.5
  circle A36 centre (51.2451, -46.0409) radius 2.5
  line L43 (-51.2451, -46.0409) -> (-52.4951, -43.8758)
  line L44 (-65.4951, -21.3591) -> (-64.2451, -23.5242)
  line L45 (-64.2451, -23.5242) -> (-72.2433, -28.142)
  line L46 (-52.4951, -43.8758) -> (-61.1551, -48.8757)
  line L47 (-65.2983, -37.7) -> (-71.1733, -27.5242)
  line L48 (-65.2983, -37.7) -> (-59.4233, -47.8758)
  line L49 (-57.7353, 37.5827) -> (-55.9675, 39.3505)
  line L50 (-37.5827, 57.7353) -> (-39.3505, 55.9675)
  line L51 (-39.3505, 55.9675) -> (-46.2035, 62.8205)
  line L52 (-55.9675, 39.3505) -> (-63.0348, 46.4178)
  line L53 (-53.3159, 53.3159) -> (-61.6244, 45.0073)
  line L54 (-53.3159, 53.3159) -> (-45.0073, 61.6244)
  line L55 (37.5827, 57.7353) -> (39.3505, 55.9675)
  line L56 (57.7353, 37.5827) -> (55.9675, 39.3505)
  line L57 (39.3505, 55.9675) -> (48.2854, 64.9024)
  line L58 (55.9675, 39.3505) -> (64.8318, 48.2147)
  line L59 (53.3159, 53.3159) -> (45.0073, 61.6244)
  line L60 (53.3159, 53.3159) -> (61.6244, 45.0073)
  line L61 (65.4951, -21.3591) -> (64.2451, -23.5242)
  line L62 (51.2451, -46.0409) -> (52.4951, -43.8758)
  line L63 (52.4951, -43.8758) -> (61.8256, -49.2628)
  line L64 (64.2451, -23.5242) -> (73.0139, -28.5869)
  line L65 (65.2983, -37.7) -> (71.1733, -27.5242)
  line L66 (65.2983, -37.7) -> (59.4233, -47.8758)
  circle A37 centre (0, 0) radius 50
  line L67 (64.2451, -23.5242) -> (47.9636, -14.1241)
  line L68 (52.4951, -43.8758) -> (36.2136, -34.4757)
  line L69 (-52.4951, -43.8758) -> (-36.2136, -34.4757)
  line L70 (-64.2451, -23.5242) -> (-47.9636, -14.1241)
  line L71 (-39.3505, 55.9675) -> (-26.0567, 42.6737)
  line L72 (-55.9675, 39.3505) -> (-42.6737, 26.0567)
  line L73 (39.3505, 55.9675) -> (26.0567, 42.6737)
  line L74 (55.9675, 39.3505) -> (42.6737, 26.0567)
  line L75 (-65.4951, -21.3591) -> (-66.7451, -19.1941)
  line L76 (-66.7451, -19.1941) -> (-49.1742, -9.0495)
  line L77 (-51.2451, -46.0409) -> (-49.9951, -48.2059)
  line L78 (-49.9951, -48.2059) -> (-32.4242, -38.0614)
  line L79 (51.2451, -46.0409) -> (49.9951, -48.2059)
  line L80 (49.9951, -48.2059) -> (32.4242, -38.0614)
  line L81 (65.4951, -21.3591) -> (66.7451, -19.1941)
  line L82 (66.7451, -19.1941) -> (49.1742, -9.0495)
  line L83 (57.7353, 37.5827) -> (59.503, 35.815)
  line L84 (59.503, 35.815) -> (45.1565, 21.4684)
  line L85 (37.5827, 57.7353) -> (35.815, 59.503)
  line L86 (35.815, 59.503) -> (21.4684, 45.1565)
  line L87 (-37.5827, 57.7353) -> (-35.815, 59.503)
  line L88 (-35.815, 59.503) -> (-21.4684, 45.1565)
  line L89 (-57.7353, 37.5827) -> (-59.503, 35.815)
  line L90 (-59.503, 35.815) -> (-45.1565, 21.4684)
  line L91 (-75, -4) -> (-75, -9)
  line L92 (-75, -9) -> (-49.1742, -9.0495)
  line L93 (-71.1733, -27.5242) -> (-81.8759, -8.9868)
  line L94 (-81.8759, -8.9868) -> (-75, -9)
  line L95 (-66.7451, -19.1941) -> (-73.6733, -23.1941)
  line L96 (75, -4) -> (75, -9)
  line L97 (75, -9) -> (49.1742, -9.0495)
  line L98 (71.1733, -27.5242) -> (81.8683, -9)
  line L99 (81.8683, -9) -> (75, -9)
  line L100 (66.7451, -19.1941) -> (73.6733, -23.1941)
  line L101 (-30.0561, -50) -> (-30.0561, -45)
  line L102 (-30.0561, -45) -> (-21.7945, -45)
  line L103 (-30.0561, -45) -> (-44.4423, -45)
  line L104 (25, -51) -> (25, -45)
  line L105 (25, -45) -> (21.7945, -45)
  line L106 (25, -45) -> (44.4423, -45)
  dimension "d84" = 5
  dimension "d85" = 5
  dimension "d86" = 5
  dimension "d87" = 5
  dimension "d88" = 5
  dimension "d89" = 5
  dimension "d90" = 5
  dimension "d91" = 5
  dimension "d92" = 5
  dimension "d93" = 5
  dimension "d94" = 5
  dimension "d95" = 5
  dimension "d96" = 5
  dimension "d97" = 6
  constraint midpoint L33 L39.start
  constraint perpendicular L33 L39
  constraint midpoint L30 L40.start
  constraint perpendicular L30 L40
  constraint midpoint L27 L41.start
  constraint perpendicular L27 L41
  constraint midpoint L24 L42.start
  constraint perpendicular L24 L42
  constraint concentric A16 A29
  constraint concentric A18 A30
  constraint concentric A19 A31
  constraint concentric A20 A32
  constraint concentric A21 A33
  constraint concentric A22 A34
  constraint concentric A23 A35
  constraint concentric A17 A36
  constraint coincident A16.centre A29.centre
  constraint coincident A29 L43.end
  constraint perpendicular L39 L43
  constraint coincident A18.centre A30.centre
  constraint coincident A30 L44.end
  constraint parallel L43 L44
  constraint tangent A30 L45
  constraint tangent A29 L46
  constraint coincident L45 L47.end
  constraint perpendicular L45 L47
  constraint coincident L46 L48.end
  constraint perpendicular L46 L48
  constraint coincident A19.centre A31.centre
  constraint coincident A31 L49.end
  constraint parallel L30 L49
  constraint coincident A20.centre A32.centre
  constraint coincident A32 L50.end
  constraint parallel L49 L50
  constraint tangent A32 L51
  constraint tangent A31 L52
  constraint coincident L52 L53.end
  constraint perpendicular L52 L53
  constraint coincident L51 L54.end
  constraint perpendicular L51 L54
  constraint coincident A21.centre A33.centre
  constraint coincident A33 L55.end
  constraint perpendicular L54 L55
  constraint coincident A22.centre A34.centre
  constraint coincident A34 L56.end
  constraint parallel L55 L56
  constraint tangent A33 L57
  constraint tangent A34 L58
  constraint coincident L57 L59.end
  constraint perpendicular L57 L59
  constraint coincident L58 L60.end
  constraint perpendicular L58 L60
  constraint coincident A23.centre A35.centre
  constraint coincident A35 L61.end
  constraint perpendicular L42 L61
  constraint coincident A17.centre A36.centre
  constraint coincident A36 L62.end
  constraint parallel L61 L62
  constraint tangent A36 L63
  constraint tangent A35 L64
  constraint coincident L64 L65.end
  constraint perpendicular L64 L65
  constraint coincident L63 L66.end
  constraint perpendicular L63 L66
  constraint concentric A0 A37
  constraint coincident A37 L67.end
  constraint tangent A35 L67
  constraint coincident A37 L68.end
  constraint tangent A36 L68
  constraint coincident A37 L69.end
  constraint tangent A29 L69
  constraint coincident A37 L70.end
  constraint tangent A30 L70
  constraint coincident A37 L71.end
  constraint tangent A32 L71
  constraint coincident A37 L72.end
  constraint tangent A31 L72
  constraint coincident A37 L73.end
  constraint tangent A33 L73
  constraint coincident A37 L74.end
  constraint tangent A34 L74
  constraint coincident A30 L75.end
  constraint parallel L44 L75
  constraint coincident A37 L76.end
  constraint tangent A30 L76
  constraint coincident A29 L77.end
  constraint perpendicular L76 L77
  constraint coincident A37 L78.end
  constraint tangent A29 L78
  constraint coincident A36 L79.end
  constraint parallel L62 L79
  constraint coincident A37 L80.end
  constraint tangent A36 L80
  constraint coincident A35 L81.end
  constraint perpendicular L80 L81
  constraint coincident A37 L82.end
  constraint tangent A35 L82
  constraint coincident A34 L83.end
  constraint parallel L56 L83
  constraint coincident A37 L84.end
  constraint tangent A34 L84
  constraint coincident A33 L85.end
  constraint perpendicular L84 L85
  constraint coincident A37 L86.end
  constraint tangent A33 L86
  constraint coincident A32 L87.end
  constraint parallel L50 L87
  constraint coincident A37 L88.end
  constraint tangent A32 L88
  constraint coincident A31 L89.end
  constraint perpendicular L88 L89
  constraint coincident A37 L90.end
  constraint tangent A31 L90
  constraint coincident L20 L91.start
  constraint perpendicular L20 L91
  constraint perpendicular L45 L93
  constraint parallel L92 L94
  constraint coincident L93 L95.end
  constraint tangent A30 L95
  constraint coincident L1 L96.start
  constraint perpendicular L1 L96
  constraint perpendicular L64 L98
  constraint perpendicular L96 L99
  constraint coincident L98 L100.end
  constraint tangent A35 L100
  constraint coincident L9 L101.start
  constraint perpendicular L9 L101
  constraint coincident A37 L102.end
  constraint perpendicular L101 L102
  constraint coincident L78 L103.end
  constraint perpendicular L101 L103
  constraint perpendicular L5 L104
  constraint coincident A37 L105.end
  constraint perpendicular L104 L105
  constraint coincident L80 L106.end
  constraint perpendicular L104 L106
  measures "d84" distance of L39.start L39.end
  measures "d85" distance of L40.start L40.end
  measures "d86" distance of L41.start L41.end
  measures "d87" distance of L42.start L42.end
  measures "d88" diameter of A29
  measures "d89" diameter of A30
  measures "d90" diameter of A31
  measures "d91" diameter of A32
  measures "d92" diameter of A33
  measures "d93" diameter of A34
  measures "d94" diameter of A35
  measures "d95" diameter of A36
  measures "d96" distance of L101.start L101.end
  measures "d97" distance of L104.start L104.end
extrude "押し出し23" cut sketch "スケッチ24" against normal blind 30 contours L57 L58 L59 L60 A37 L73 L74 | L82 L97 L98 L99 L100 | L63 L64 L65 L66 A37 L67 L68 | A37 L80 L105 L106 | L51 L52 L53 L54 A37 L71 L72 | A37 L78 L102 L103 | L45 L46 L47 L48 A37 L69 L70 | L76 L92 L93 L94 L95 bodies 1